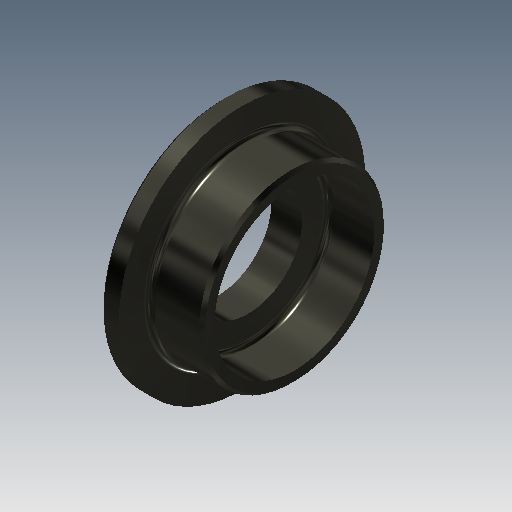
# Autodesk Inventor part: CoverOutput
Saved by Autodesk Inventor 2020.1 (Build 241239000, 239)
## iProperties
Shininess: 64.0
Length Units: 11269
Angle Units: 11279
Time Units: 11290
Mass Units: 11283
Length Display Precision: 3
Angle Display Precision: 2
Compacted: True
Part Number: CoverOutput
Document SubType Name: Modeling
Created: 2003-11-06
Designer: ales
Manufacturer: Standard
Standards Organization: Custom
Material: Generic
Density: 1 g/cm^3
Appearance: Gunmetal
Density: 0.0
Volumn: 0.0
Area: 0.0
PropertySet Name: Model Information
Control State: 0
Master: False
Checked Out: False
Author: ales
Autodesk Inventor part; units mm, degrees
ref_plane "YZ Plane" through (0, 0, 0) normal (1, 0, 0) x (0, 1, 0)
ref_plane "XZ Plane" through (0, 0, 0) normal (0, 1, 0) x (-1, 0, 0)
ref_plane "XY Plane" through (0, 0, 0) normal (0, 0, 1) x (1, 0, 0)
sketch "Sketch1" plane through (0, 0, 0) normal (0, 0, 1) x (1, 0, 0)
  line L0 (0, 0) -> (23.0859, 0)
  line L1 (0, 17.5) -> (10, 17.5)
  line L2 (10, 17.5) -> (10, 26)
  line L3 (10, 26) -> (25, 26)
  line L4 (0, 22.5) -> (0, 17.5)
  line L5 (2, 22.5) -> (2, 40)
  line L6 (2, 40) -> (8, 40)
  line L7 (8, 40) -> (8, 30)
  line L8 (8, 30) -> (25, 30)
  line L9 (25, 30) -> (25, 26)
  line L10 (0, 22.5) -> (2, 22.5)
  dimension "d0" = 35
  dimension "d1" = 52
  dimension "d2" = 15
  dimension "d3" = 6
  dimension "d4" = 80
  dimension "d5" = 60
  dimension "d6" = 45
  dimension "d7" = 25
  dimension "d8" = 8
  constraints: 22 end point, 6 perpendicular, 1 horizontal, 1 parallel, 1 point on line, 1 vertical, 1 other
  measures "d0" diameter of L1 L0
  measures "d1" diameter of L3 L0
  measures "d2" distance of L2.end L3.end
  measures "d3" distance of L5.end L6.end
  measures "d4" diameter of L6 L0
  measures "d5" diameter of L8 L0
  measures "d6" diameter of L10 L0
  measures "d7" distance between parallel lines of L9 L4
  measures "d8" distance between parallel lines of L4 L7
revolve "Revolution1" add sketch "Sketch1" angle 360 about axis through (0, 0, 0) along (1, 0, 0)
fillet "Fillet1" radius 2 3 edges at (2, -22.5, 0) (8, -30, 0) (10, -26, 0)
chamfer "Chamfer1" distance 1 angle 45 2 edges at (25, -30, 0) (2, -40, 0)
body "Solid1"
